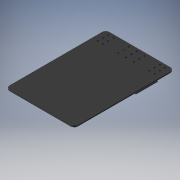
# Autodesk Inventor part: Sensor Calibration Rail Carriage
Saved by Autodesk Inventor 2019 (Build 230136000, 136)
## iProperties
Created: 2019-01-19
Part Number: Sensor Calibration Rail Carriage
Material: Generic
Document SubType Name: Modeling
Designer: Billy
Density: 1 g/cm^3
Appearance: Default
Author: Billy
Autodesk Inventor part; units mm, degrees
ref_plane "YZ Plane" through (0, 0, 0) normal (1, 0, 0) x (0, 1, 0)
ref_plane "XZ Plane" through (0, 0, 0) normal (0, 1, 0) x (-1, 0, 0)
ref_plane "XY Plane" through (0, 0, 0) normal (0, 0, 1) x (1, 0, 0)
sketch "Sketch1" plane through (0, 0, 0) normal (0, 0, 1) x (1, 0, 0)
  line L0 (0, 0) -> (50, 0) construction
  line L1 (0, 0) -> (-4.2426, -4.2426)
  line L2 (0, 0) -> (6, 0) construction
  line L3 (0, 0) -> (4.2426, -4.2426)
  line L4 (0, 0) -> (6, 0) construction
  line L5 (50, 0) -> (45.7574, -4.2426)
  line L6 (50, 0) -> (54.2426, -4.2426)
  line L7 (0, 0) -> (37, 0) construction
  line L8 (-4.2426, -4.2426) -> (-7.0711, -1.4142)
  line L9 (-7.0711, -1.4142) -> (-3, 2.6569)
  line L10 (3, 2.6569) -> (7.0711, -1.4142)
  line L11 (7.0711, -1.4142) -> (4.2426, -4.2426)
  line L12 (3, 2.6569) -> (3, 36)
  line L13 (3, 5.6569) -> (3, 36)
  line L14 (-3, 36) -> (-3, 2.6569)
  line L15 (45.7574, -4.2426) -> (42.9289, -1.4142)
  line L16 (42.9289, -1.4142) -> (47, 2.6569)
  line L17 (53, 2.6569) -> (57.0711, -1.4142)
  line L18 (57.0711, -1.4142) -> (54.2426, -4.2426)
  line L19 (53, 2.6569) -> (53, 36)
  line L20 (47, 36) -> (47, 2.6569)
  line L21 (3, 36) -> (47, 36)
  line L22 (53, 36) -> (53, 42)
  line L23 (53, 42) -> (-3, 42)
  line L24 (-3, 42) -> (-3, 36)
  dimension "d2" = 6
  dimension "d4" = 6
  dimension "d6" = 6
  dimension "d7" = 6
  dimension "d11" = 4
  dimension "d12" = 90
  dimension "d17" = 4
  dimension "d18" = 90
  constraints: 50 end point, 5 horizontal, 5 perpendicular, 3 parallel, 2 equal length
  measures "d2" distance of L0.start L1.end
  measures "d4" distance of L0.start L3.end
  measures "d6" distance of L5.end L0.end
  measures "d7" distance of L6.end L0.end
  measures "d11" distance of L1.end L8.end
  measures "d12" angle of L8 L9
  measures "d17" distance of L5.end L15.end
  measures "d18" angle of L15 L16
extrude "Extrusion1" add sketch "Sketch1" along normal blind 40
move faces "Move1" translate (5, 0, 0) faces at (53, 40, 13.3333) (53, 24.8856, 13.3333) (54.357, 1.2998, 13.3333) (47, 13.7712, 13.3333) (44.286, -0.0572, 26.6667) (52.8284, -2.8284, 13.3333) (48.5858, -1.4142, 13.3333) (56.1283, -2.357, 13.3333) (44.8146, -3.2998, 13.3333)
sketch "Sketch2" plane through (0, 0, 40) normal (0, 0, 1) x (1, 0, 0)
  line L0 (-4.2426, -4.2426) -> (0, 0) projected
  line L1 (0, 0) -> (4.2426, -4.2426) projected
  line L2 (4.2426, -4.2426) -> (7.0711, -1.4142) projected
  line L3 (7.0711, -1.4142) -> (3, 2.6569) projected
  line L4 (3, 2.6569) -> (3, 36) projected
  line L5 (3, 36) -> (52, 36) projected
  line L6 (52, 36) -> (52, 2.6569) projected
  line L7 (52, 2.6569) -> (47.9289, -1.4142) projected
  line L8 (47.9289, -1.4142) -> (50.7574, -4.2426) projected
  line L9 (50.7574, -4.2426) -> (55, 0) projected
  line L10 (55, 0) -> (59.2426, -4.2426) projected
  line L11 (59.2426, -4.2426) -> (62.0711, -1.4142) projected
  line L12 (62.0711, -1.4142) -> (58, 2.6569) projected
  line L13 (58, 2.6569) -> (58, 42) projected
  line L14 (58, 42) -> (-3, 42) projected
  line L15 (-3, 42) -> (-3, 2.6569) projected
  line L16 (-3, 2.6569) -> (-7.0711, -1.4142) projected
  line L17 (-7.0711, -1.4142) -> (-4.2426, -4.2426) projected
  circle A0 centre (0, -3.5355) radius 2.5
  line L18 (0, 0) -> (4.2426, -4.2426) projected
  line L19 (-4.2426, -4.2426) -> (0, 0) projected
  line L20 (2.5, -3.5355) -> (2.5, 6.4645)
  line L21 (2.5, -3.5355) -> (12.5, -3.5355) construction
  circle A1 centre (27.5, 6.4645) radius 5.25
  line L22 (52, 17.1716) -> (3, 17.1716)
  line L23 (50.7574, -4.2426) -> (4.2426, -4.2426)
  dimension "d25" = 5
  dimension "d26" = 10
  dimension "d27" = 90
  dimension "d83" = 10.5
  constraints: 8 end point, 3 point on line, 2 horizontal, 1 centre point, 1 horizontal alignment, 1 perpendicular, 1 vertical, 4 other
  measures "d26" distance of L20.start L20.end
  measures "d27" angle of L21 L20
  measures "d83" diameter of A1
extrude "Extrusion2" add sketch "Sketch2" against normal blind 5 contours L2 L3 L4 L22 L6 L7 L8 L23
sketch "Sketch4" plane through (-3, 42, 40) normal (0, 1, 0) x (1, 0, 0)
  line L0 (0, 40) -> (61, 40) projected
  line L1 (0, 40) -> (0, 0) projected
  line L2 (61, 0) -> (0, 0) projected
  line L3 (61, 40) -> (61, 0) projected
  line L4 (-19.5, 0) -> (-19.5, -150)
  line L5 (-19.5, -150) -> (30.5, -150)
  line L6 (80.5, 0) -> (80.5, -150)
  line L7 (80.5, -150) -> (30.5, -150)
  line L8 (61, 40) -> (80.5, 40)
  line L9 (80.5, 40) -> (80.5, 0)
  line L10 (61, 0) -> (61, 40)
  line L11 (0, 40) -> (-19.5, 40)
  line L12 (-19.5, 40) -> (-19.5, 0)
  line L13 (0, 0) -> (0, 40)
  point P0 (3, 40)
  dimension "d58" = 50
  dimension "d59" = 150
  dimension "d60" = 50
  constraints: 20 end point, 2 horizontal, 2 parallel, 2 perpendicular, 1 point on line
  measures "d58" distance of L5.end L4.end
  measures "d59" distance of L4.end L4.start
  measures "d60" distance of L6.end L5.end
extrude "Extrusion4" add sketch "Sketch4" against normal blind 2.5 contours L1 L2 L3 L8 L9 L6 L7 L5 L4 L12 L11
sketch "Sketch5" plane through (0, 0, 40) normal (0, 0, 1) x (1, 0, 0)
  line L0 (58, 39.5) -> (-3, 39.5) projected
  line L1 (-3, 39.5) -> (-3, 2.6569) projected
  line L2 (-3, 2.6569) -> (-7.0711, -1.4142) projected
  line L3 (-7.0711, -1.4142) -> (-4.2426, -4.2426) projected
  line L4 (-4.2426, -4.2426) -> (0, 0) projected
  line L5 (0, 0) -> (4.2426, -4.2426) projected
  line L6 (4.2426, -4.2426) -> (50.7574, -4.2426) projected
  line L7 (50.7574, -4.2426) -> (55, 0) projected
  line L8 (55, 0) -> (59.2426, -4.2426) projected
  line L9 (59.2426, -4.2426) -> (62.0711, -1.4142) projected
  line L10 (62.0711, -1.4142) -> (58, 2.6569) projected
  line L11 (58, 2.6569) -> (58, 39.5) projected
  circle A0 centre (27.5, 6.4645) radius 5.25 projected
  line L12 (52, 17.1716) -> (3, 17.1716) projected
  line L13 (3, 17.1716) -> (3, 36) projected
  line L14 (3, 36) -> (52, 36) projected
  line L15 (52, 36) -> (52, 17.1716) projected
  circle A1 centre (0, -3.5355) radius 2.5
  line L16 (0, 0) -> (4.2426, -4.2426) projected
  line L17 (-4.2426, -4.2426) -> (0, 0) projected
  line L18 (0, -3.5355) -> (0, 31.4645)
  dimension "d63" = 5
  dimension "d64" = 35
  constraints: 2 end point, 2 tangent, 1 centre point, 1 parallel
  measures "d63" diameter of A1
  measures "d64" distance of L18.start L18.end
move faces "Move2" translate (0, -8.0355, 0) faces at (37.6667, 39.5, 140) (35.6667, 36, 13.3333) (10.8333, 42, 63.3333)
move faces "Move3" translate (-15, 0, 0) faces at (-22.5, 33.1311, 63.3333)
move faces "Move4" translate (15, 0, 0) faces at (77.5, 33.1311, 126.6667)
sketch "Sketch6" plane through (0, 0, 40) normal (0, 0, 1) x (1, 0, 0)
  line L0 (58, 31.4645) -> (-3, 31.4645) projected
  line L1 (-3, 31.4645) -> (-3, 2.6569) projected
  line L2 (-3, 2.6569) -> (-7.0711, -1.4142) projected
  line L3 (-7.0711, -1.4142) -> (-4.2426, -4.2426) projected
  line L4 (-4.2426, -4.2426) -> (0, 0) projected
  line L5 (0, 0) -> (4.2426, -4.2426) projected
  line L6 (4.2426, -4.2426) -> (50.7574, -4.2426) projected
  line L7 (50.7574, -4.2426) -> (55, 0) projected
  line L8 (55, 0) -> (59.2426, -4.2426) projected
  line L9 (59.2426, -4.2426) -> (62.0711, -1.4142) projected
  line L10 (62.0711, -1.4142) -> (58, 2.6569) projected
  line L11 (58, 2.6569) -> (58, 31.4645) projected
  circle A0 centre (27.5, 6.4645) radius 5.25 projected
  line L12 (52, 17.1716) -> (3, 17.1716) projected
  line L13 (3, 17.1716) -> (3, 27.9645) projected
  line L14 (3, 27.9645) -> (52, 27.9645) projected
  line L15 (52, 27.9645) -> (52, 17.1716) projected
  line L16 (27.5, 6.4645) -> (33.1569, 12.1213)
  line L17 (27.5, 6.4645) -> (35.5, 6.4645) construction
  circle A1 centre (33.1569, 12.1213) radius 2
  circle A2 centre (21.8431, 12.1213) radius 2
  circle A3 centre (21.8431, 0.8076) radius 2
  circle A4 centre (33.1569, 0.8076) radius 2
  dimension "d74" = 8
  dimension "d75" = 45
  dimension "d76" = 4
  dimension "d79" = 360
  constraints: 4 centre point, 4 end point, 1 coincident, 1 equal length, 1 horizontal, 9 other
  measures "d74" distance of L16.start L16.end
  measures "d75" angle of L17 L16
  measures "d76" diameter of A1
extrude "Extrusion5" cut sketch "Sketch6" against normal up to surface (5 mm away) contours A1 | A2 | A3 | A4
sketch "Sketch8" plane through (0, 0, 40) normal (0, 0, 1) x (1, 0, 0)
  circle A0 centre (21.8431, 0.8076) radius 2 projected
  circle A1 centre (33.1569, 0.8076) radius 2 projected
  circle A2 centre (21.8431, 12.1213) radius 2 projected
  circle A3 centre (33.1569, 12.1213) radius 2 projected
  line L0 (58, 31.4645) -> (-3, 31.4645) projected
  line L1 (-3, 31.4645) -> (-3, 2.6569) projected
  line L2 (-3, 2.6569) -> (-7.0711, -1.4142) projected
  line L3 (-7.0711, -1.4142) -> (-4.2426, -4.2426) projected
  line L4 (-4.2426, -4.2426) -> (0, 0) projected
  line L5 (0, 0) -> (4.2426, -4.2426) projected
  line L6 (4.2426, -4.2426) -> (50.7574, -4.2426) projected
  line L7 (50.7574, -4.2426) -> (55, 0) projected
  line L8 (55, 0) -> (59.2426, -4.2426) projected
  line L9 (59.2426, -4.2426) -> (62.0711, -1.4142) projected
  line L10 (62.0711, -1.4142) -> (58, 2.6569) projected
  line L11 (58, 2.6569) -> (58, 31.4645) projected
  circle A4 centre (27.5, 6.4645) radius 5.25 projected
  line L12 (52, 17.1716) -> (3, 17.1716) projected
  line L13 (3, 17.1716) -> (3, 27.9645) projected
  line L14 (3, 27.9645) -> (52, 27.9645) projected
  line L15 (52, 27.9645) -> (52, 17.1716) projected
  line L16 (33.1569, -3.1924) -> (21.8431, -3.1924)
  line L17 (17.8431, 0.8076) -> (17.8431, 12.1213)
  line L18 (21.8431, 16.1213) -> (33.1569, 16.1213)
  line L19 (37.1569, 12.1213) -> (37.1569, 0.8076)
  arc A5 (25.7822, 1.5035) -> (22.539, 4.7466) centre (21.8431, 0.8076) ccw
  arc A6 (17.8431, 0.8076) -> (21.8431, -3.1924) centre (21.8431, 0.8076) ccw
  arc A7 (33.1569, -3.1924) -> (37.1569, 0.8076) centre (33.1569, 0.8076) ccw
  arc A8 (32.461, 4.7466) -> (29.2178, 1.5035) centre (33.1569, 0.8076) ccw
  arc A9 (37.1569, 12.1213) -> (33.1569, 16.1213) centre (33.1569, 12.1213) ccw
  arc A10 (29.2178, 11.4255) -> (32.461, 8.1823) centre (33.1569, 12.1213) ccw
  arc A11 (21.8431, 16.1213) -> (17.8431, 12.1213) centre (21.8431, 12.1213) ccw
  arc A12 (22.539, 8.1823) -> (25.7822, 11.4255) centre (21.8431, 12.1213) ccw
  constraints: 16 point on circle, 8 centre point, 8 end point, 4 coincident, 2 parallel, 1 horizontal, 1 perpendicular, 9 other
extrude "Extrusion6" cut sketch "Sketch8" against normal blind 4 contours L16 A6 L17 A11 L18 A9 L19 A7
move faces "Move5" translate (0, 0, -4) faces at (46.3662, 10.4904, 35)
move faces "Move6" translate (0, 14.2929, 0) faces at (35.6667, 17.1716, 37)
fillet "Fillet1" radius 7 4 edges at (-37.5, 32.7145, 0) (92.5, 32.7145, 0) (92.5, 32.7145, 190) (-37.5, 32.7145, 190)
fillet "Fillet2" radius 1 4 edges at (-7.0711, -1.4142, 20) (-4.2426, -4.2426, 20) (59.2426, -4.2426, 20) (62.0711, -1.4142, 20)
fillet "Fillet3" radius 1 4 edges at (50.7574, -4.2426, 15.5) (47.9289, -1.4142, 15.5) (7.0711, -1.4142, 15.5) (4.2426, -4.2426, 15.5)
fillet "Fillet4" radius 2 2 edges at (50.7574, -4.2426, 35.5) (4.2426, -4.2426, 35.5)
sketch "Sketch9" plane through (-3, 31.4645, 40) normal (0, -1, 0) x (1, 0, 0)
  line L0 (55, -9) -> (6, -9) projected
  line L1 (6, -40) -> (6, -9) projected
  line L2 (55, -40) -> (6, -40) projected
  line L3 (55, -40) -> (55, -9) projected
  arc A0 (-27.5, 150) -> (-34.5, 143) centre (-27.5, 143) ccw projected
  line L4 (-34.5, 143) -> (-34.5, -33) projected
  arc A1 (-34.5, -33) -> (-27.5, -40) centre (-27.5, -33) ccw projected
  line L5 (-27.5, -40) -> (0, -40) projected
  line L6 (0, 0) -> (0, -40) projected
  line L7 (61, 0) -> (0, 0) projected
  line L8 (61, -40) -> (61, 0) projected
  line L9 (61, -40) -> (88.5, -40) projected
  arc A2 (88.5, -40) -> (95.5, -33) centre (88.5, -33) ccw projected
  line L10 (95.5, -33) -> (95.5, 143) projected
  arc A3 (95.5, 143) -> (88.5, 150) centre (88.5, 143) ccw projected
  line L11 (88.5, 150) -> (-27.5, 150) projected
  circle A4 centre (30.5, -24.5) radius 2
  circle A5 centre (30.5, -34.5) radius 2
  circle A6 centre (30.5, -14.5) radius 2
  circle A7 centre (15.5, -34.5) radius 2
  circle A8 centre (15.5, -24.5) radius 2
  circle A9 centre (15.5, -14.5) radius 2
  circle A10 centre (45.5, -34.5) radius 2
  circle A11 centre (45.5, -24.5) radius 2
  circle A12 centre (45.5, -14.5) radius 2
  circle A13 centre (74.75, -24.5) radius 2
  circle A14 centre (74.75, -14.5) radius 2
  circle A15 centre (84.75, -24.5) radius 2
  circle A16 centre (84.75, -14.5) radius 2
  circle A17 centre (74.75, -34.5) radius 2
  circle A18 centre (84.75, -34.5) radius 2
  line L12 (30.5, -34.5) -> (30.5, -14.5)
  circle A19 centre (-13.75, -24.5) radius 2
  circle A20 centre (-13.75, -14.5) radius 2
  circle A21 centre (-23.75, -24.5) radius 2
  circle A22 centre (-23.75, -14.5) radius 2
  circle A23 centre (-13.75, -34.5) radius 2
  circle A24 centre (-23.75, -34.5) radius 2
  point P0 (3, -40)
  dimension "d100" = 4
  dimension "d103" = 10
  dimension "d110" = 10
  dimension "d120" = 15
  dimension "d124" = 15
  dimension "d129" = 4
  dimension "d132" = 10
  dimension "d135" = 10
  dimension "d140" = 10
  constraints: 21 centre point, 6 symmetric about line, 5 vertical, 3 horizontal, 2 end point, 32 other
  measures "d100" diameter of A4
  measures "d103" distance of A4.centre L12.start
  measures "d110" distance of A4.centre L12.end
  measures "d120" distance of L12.start A7.centre
  measures "d124" distance of L12.start A10.centre
  measures "d129" diameter of A13
  measures "d132" distance of A13.centre A14.centre
  measures "d135" distance of A13.centre A15.centre
  measures "d140" distance of A13.centre A17.centre
extrude "Extrusion7" cut sketch "Sketch9" against normal up to surface (6 mm away) from surface at 3.5 contours A4 L12 | L12 A4 | A5 | A6 | A7 | A8 | A9 | A10 | A11 | A12 | A13 | A14 | A15 | A16 | A17 | A18 | A19 | A20 | A21 | A22 | A23 | A24
body "Solid1"
